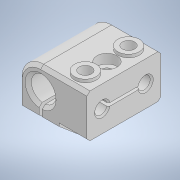
# Autodesk Inventor part: XY Joiner
Saved by Autodesk Inventor 2022 (Build 260153000, 153)
## iProperties
Created: 2022-04-23
Part Number: XY Joiner
Material: Generic
Document SubType Name: Modeling
Designer: Nick
Density: 1 g/cm^3
Appearance: Default
Author: Nick
Autodesk Inventor part; units mm, degrees
ref_plane "YZ Plane" through (0, 0, 0) normal (1, 0, 0) x (0, 1, 0)
ref_plane "XZ Plane" through (0, 0, 0) normal (0, 1, 0) x (-1, 0, 0)
ref_plane "XY Plane" through (0, 0, 0) normal (0, 0, 1) x (1, 0, 0)
sketch "Sketch1" plane through (0, 0, 0) normal (0, 0, 1) x (1, 0, 0)
  line L0 (0, 14) -> (0, 11)
  line L1 (0, 14) -> (15, 14)
  line L2 (15, 14) -> (15, 0)
  circle A0 centre (0, 7) radius 4
  line L3 (0, 3) -> (0, 0) construction
  line L4 (0, 0) -> (15, 0)
  line L5 (0, 11) -> (0, 3) construction
  line L6 (0.5, 0) -> (-0.5, 0)
  line L7 (-0.5, 0) -> (-0.5, 3.0314)
  line L8 (-0.5, 3.0314) -> (0.5, 3.0314)
  line L9 (0.5, 3.0314) -> (0.5, 0)
  line L10 (-0.5, 0) -> (-7, 0)
  line L11 (-7, 0) -> (-7, 14)
  line L12 (-7, 14) -> (0, 14)
  line L13 (-4, 10.1012) -> (-4, 3.4286) construction
  point P0 (0, 3.0314)
  dimension "d0" = 8
  dimension "d1" = 15
  dimension "d2" = 14
  dimension "d79" = 1
  dimension "d80" = 3
  dimension "d81" = 3
  constraints: 28 end point, 5 horizontal, 4 vertical, 3 perpendicular, 2 coincident, 2 midpoint, 2 parallel, 2 point on circle, 2 point on line, 1 centre point, 1 collinear, 1 tangent
  measures "d0" diameter of A0
  measures "d1" distance of L0.start L1.end
  measures "d2" distance between parallel lines of L4 L1
  measures "d79" distance of L7.end L8.end
  measures "d80" distance of L3.start L3.end
  measures "d81" distance between parallel lines of L13 L11
extrude "Extrusion1" add sketch "Sketch1" along normal blind 24 contours L1 L2 L4 L9 A0 L0 | L0 A0 L7 L10 L11 L12
sketch "Sketch2" plane through (15, 0, 0) normal (1, 0, 0) x (0, 0, -1)
  line L0 (-24, 0) -> (-24, 14) projected
  line L1 (0, 0) -> (0, 14) projected
  point P0 (-19, 7)
  point P1 (-5, 7)
  point P2 (-24, 7)
  dimension "d5" = 5
  dimension "d6" = 5
  dimension "d7" = 14
  constraints: 2 horizontal alignment, 1 midpoint
  measures "d5" distance of point (-24, 7) point (-19, 7)
  measures "d6" distance from line of L1 point (-5, 7)
  measures "d7" distance of point (-5, 7) point (-19, 7)
hole "Hole1" at (15, 7, 19) at (15, 7, 5) direction (-1, 0, 0) diameter 4 depth 10
sketch "Sketch4" plane through (0, 14, 0) normal (0, 1, 0) x (1, 0, 0)
  circle A0 centre (9.5, -5) radius 3.5
  circle A1 centre (9.5, -19) radius 3.5
  line L0 (15, -24) -> (-7, -24) projected
  line L1 (15, 0) -> (0, 0) projected
  line L2 (-0.5, 0) -> (0.5, 0) projected
  line L3 (-0.5, -24) -> (0.5, -24) projected
  line L4 (4, -24) -> (4, 0) projected
  line L5 (4, -24) -> (4, 0)
  line L6 (4, -24) -> (4, 0) projected
  line L7 (15, 0) -> (15, -24) projected
  line L8 (0.5, 0) -> (0.5, -24) projected
  line L9 (-0.5, 0) -> (-0.5, -24) projected
  point P0 (4, -24)
  point P1 (0, -24)
  dimension "d18" = 7
  dimension "d19" = 7
  dimension "d20" = 14
  dimension "d21" = 5
  dimension "d22" = 5
  dimension "d42" = 5.5
  dimension "d43" = 5.5
  constraints: 3 point on line, 2 centre point, 2 end point, 2 midpoint, 1 vertical alignment
  measures "d18" diameter of A0
  measures "d19" diameter of A1
  measures "d20" distance of A0.centre A1.centre
  measures "d21" distance from line of L0 A1.centre
  measures "d22" distance from line of A0.centre L1
  measures "d42" distance from line of L4 A1.centre
  measures "d43" distance from line of L7 A1.centre
extrude "Extrusion2" add sketch "Sketch4" along normal blind 1 contours A0 | A1
sketch "Sketch3" plane through (2, 15, 0) normal (0, 1, 0) x (1, 0, 0)
  circle A0 centre (7.5, -5) radius 3.5 projected
  circle A1 centre (7.5, -19) radius 3.5 projected
  constraints: 2 coincident, 1 vertical alignment
hole "Hole2" at (9.5, 15, 19) at (9.5, 15, 5) direction (0, -1, 0) diameter 4 depth 7
sketch "Sketch5" plane through (15, 0, 0) normal (1, 0, 0) x (0, 0, -1)
  line L0 (-17.0635, 7.5) -> (-6.9365, 7.5)
  line L1 (-6.9365, 7.5) -> (-6.9365, 6.5)
  line L2 (-6.9365, 6.5) -> (-17.0635, 6.5)
  line L3 (-17.0635, 6.5) -> (-17.0635, 7.5)
  circle A0 centre (-5, 7) radius 2 projected
  circle A1 centre (-19, 7) radius 2 projected
  point P0 (0, 0)
  point P1 (-6.9365, 7)
  point P2 (-17.0635, 6.5)
  dimension "d35" = 1
  constraints: 8 end point, 2 parallel, 1 horizontal, 1 horizontal alignment, 1 midpoint, 1 perpendicular, 4 other
  measures "d35" distance of L0.end L1.end
extrude "Extrusion3" cut sketch "Sketch5" against normal blind 8 contours L0 A0 L2 A1
sketch "Sketch6" plane through (0, 0, 0) normal (0, 0, -1) x (-1, 0, 0)
  line L0 (0, 3) -> (0, 0) projected
  arc A0 (-6, 1) -> (0, 0) centre (0, 18.5) ccw
  line L1 (-15, 0) -> (-15, 14) projected
  line L2 (-15, 2) -> (-12, 2)
  arc A1 (-6, 1) -> (-12, 2) centre (-12, -16.5) ccw
  line L3 (0, 0) -> (-15, 0) projected
  line L4 (-6, 1) -> (0, 0) construction
  line L5 (-6, 1) -> (-12, 2) construction
  dimension "d38" = 2
  dimension "d39" = 3
  constraints: 6 end point, 4 point on circle, 2 centre point, 2 tangent, 1 collinear, 1 equal radius, 1 horizontal, 1 point on line
  measures "d38" distance between parallel lines of L3 L2
  measures "d39" distance of L2.start L2.end
extrude "Extrusion4" [suppressed]
sketch "Sketch7" plane through (0, 14, 0) normal (0, 1, 0) x (1, 0, 0)
  circle A0 centre (9.5, -5) radius 2 projected
  circle A1 centre (9.5, -19) radius 2 projected
  point P0 (0, 0)
  point P1 (9.5, -12)
  dimension "d44" = 7
  dimension "d45" = 7
  constraints: 1 vertical alignment
  measures "d44" distance of A0.centre point (9.5, -12)
  measures "d45" distance of A1.centre point (9.5, -12)
hole "Hole3" at (9.5, 14, 12) direction (0, -1, 0) diameter 3.4 end through all counterbore diameter 6.5 counterbore depth 3 clearance for "Socket Head Cap Screw" size "M3" standard "Ansi Metric M Profile"
chamfer "Chamfer3" distance 0.5 angle 45 3 edges at (15, 8.9841, 4.748) (15, 5.0159, 4.748) (15, 7, 21)
ref_plane "Work Plane1" through (7, 3.5, 17.0635) normal (0, 1, 0) x (1, 0, 0)
sketch "Sketch10" plane through (7, 3.5, 17.0635) normal (0, 1, 0) x (1, 0, 0)
  circle A0 centre (2.5, 5.0635) radius 1.7 projected
  line L0 (-0.25, 3.4758) -> (-0.25, 6.6512)
  line L1 (-0.25, 6.6512) -> (2.5, 8.2389)
  line L2 (2.5, 8.2389) -> (5.25, 6.6512)
  line L3 (5.25, 6.6512) -> (5.25, 3.4758)
  line L4 (5.25, 3.4758) -> (2.5, 1.8881)
  line L5 (2.5, 1.8881) -> (-0.25, 3.4758)
  point P0 (-7, 17.0635)
  dimension "d75" = 5.5
  constraints: 12 end point, 1 coincident, 1 vertical, 13 other
  measures "d75" distance between parallel lines of L3 L0
extrude "Extrusion6" cut sketch "Sketch10" against normal blind 10
sketch "Sketch12" plane through (-0.5, 0, 0) normal (1, 0, 0) x (0, 0, -1)
  circle A0 centre (-12, -3.25) radius 1.7
  circle A1 centre (-12, -3.25) radius 5.25
  line L0 (0, 0) -> (-8.616, -7.2639)
  line L1 (-24, 0) -> (-15.384, -7.2639)
  circle A2 centre (-12, -3.25) radius 3.25
  line L2 (0, 0) -> (-24, 0) projected
  point P0 (-12, 0)
  dimension "d82" = 3.4
  dimension "d84" = 2
  dimension "d95" = 6.5
  constraints: 4 end point, 3 centre point, 3 tangent, 2 coincident, 2 point on circle, 1 midpoint, 1 vertical alignment
  measures "d82" diameter of A0
  measures "d84" radial gap between concentric circles of A1 A2
  measures "d95" diameter of A2
extrude "Extrusion7" add sketch "Sketch12" against normal blind 5.5 contours A0 | A2 | A1 L2 | L1 L2 A1 | A1 L2 L0 picked at (-14.5812, -7.0055)
ref_plane "Work Plane3" through (0, 3.0314, 24) normal (1, 0, 0) x (0, 0, -1)
mirror "Mirror1" about plane through (0, 3.0314, 24) normal (1, 0, 0) of "Extrusion7"
fillet "Fillet1" radius 7 1 edges at (-7, 14, 12)
sketch "Sketch14" plane through (6.75, 3.5, 13.5877) normal (1, 0, 0) x (0, 0, -1)
  arc A0 (-1.7963, -10.7639) -> (4.9717, -10.7639) centre (1.5877, -6.75) ccw projected
  line L0 (0, -9.5) -> (-1.5877, -6.75)
  line L1 (-1.5877, -6.75) -> (0, -4)
  line L2 (0, -4) -> (3.1754, -4)
  line L3 (3.1754, -4) -> (4.7631, -6.75)
  line L4 (4.7631, -6.75) -> (3.1754, -9.5)
  line L5 (3.1754, -9.5) -> (0, -9.5)
  point P0 (13.5877, -3.5)
  dimension "d96" = 5.5
  constraints: 12 end point, 1 coincident, 1 horizontal, 13 other
  measures "d96" distance between parallel lines of L4 L1
extrude "Extrusion8" cut sketch "Sketch14" against normal blind 2.5
sketch "Sketch13" plane through (-7, 0, 0) normal (-1, 0, 0) x (0, 0, 1)
  arc A0 (8.616, -7.2639) -> (15.384, -7.2639) centre (12, -3.25) ccw projected
  point P0 (0, 0)
  constraints: 1 coincident
hole "Hole4" at (-7, -3.25, 12) direction (1, 0, 0) diameter 3.4 end through all counterbore diameter 6.5 counterbore depth 3 clearance for "Socket Head Cap Screw" size "M3" standard "Ansi Metric M Profile"
chamfer "Chamfer5" distance 1 angle 45 11 edges at (10.5, 0, 24) (0, 11, 24) (0, 11, 0) (10.5, 0, 0) (-4.9497, 11.9497, 0) (-7, 3.5, 0) (7.5, 14, 0) (7.5, 14, 24) (-4.9497, 11.9497, 24) (-7, 3.5, 24) (-7, 0, 12)
equation "\"d81\" = d80"
equation "\"d6\" = d5"
equation "\"d22\" = d21"
equation "\"d42\" = d43"
equation "\"d44\" = d45"
body "Solid1"
